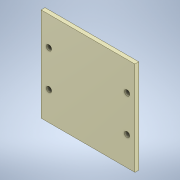
# Autodesk Inventor part: steelPlateForGate
Saved by Autodesk Inventor 2020 (Build 240168000, 168)
## iProperties
Created: 2019-07-06
Part Number: steelPlateForGate
Material: Steel, Mild
Document SubType Name: Modeling
Designer: steele
Density: 7.85 g/cm^3
Appearance: Smooth - Ash
Author: steele
Autodesk Inventor part; units mm, degrees
ref_plane "YZ Plane" through (0, 0, 0) normal (1, 0, 0) x (0, 1, 0)
ref_plane "XZ Plane" through (0, 0, 0) normal (0, 1, 0) x (-1, 0, 0)
ref_plane "XY Plane" through (0, 0, 0) normal (0, 0, 1) x (1, 0, 0)
sketch "Sketch1" plane through (0, 0, 0) normal (0, 0, 1) x (1, 0, 0)
  line L0 (-76.2, -76.2) -> (76.2, -76.2)
  line L1 (76.2, -76.2) -> (76.2, 76.2)
  line L2 (76.2, 76.2) -> (-76.2, 76.2)
  line L3 (-76.2, 76.2) -> (-76.2, -76.2)
  line L4 (-76.2, -76.2) -> (76.2, 76.2) construction
  line L5 (76.2, -76.2) -> (-76.2, 76.2) construction
  point P0 (0, 0)
  dimension "d0" = 152.4
  dimension "d1" = 152.4
  constraints: 12 end point, 2 midpoint, 2 parallel, 1 horizontal, 1 perpendicular
  measures "d0" distance of L0.start L0.end
  measures "d1" distance of L1.end L0.end
extrude "Extrusion1" add sketch "Sketch1" along normal blind 6.35
sketch "Sketch2" plane through (0, 0, 6.35) normal (0, 0, 1) x (1, 0, 0)
  line L0 (-63.5, -29.3688) -> (63.5, -29.3688) construction
  line L1 (63.5, -29.3688) -> (63.5, 29.3688) construction
  line L2 (63.5, 29.3688) -> (-63.5, 29.3687) construction
  line L3 (-63.5, 29.3687) -> (-63.5, -29.3688) construction
  line L4 (-63.5, -29.3688) -> (63.5, 29.3688) construction
  line L5 (63.5, -29.3688) -> (-63.5, 29.3687) construction
  point P0 (0, 0)
  dimension "d4" = 127
  dimension "d5" = 58.7375
  constraints: 12 end point, 4 coincident, 2 midpoint, 2 parallel, 1 horizontal, 1 perpendicular
  measures "d4" distance of L0.start L0.end
  measures "d5" distance of L2.end L0.start
hole "Hole1" at (-63.5, 29.3687, 6.35) at (63.5, 29.3688, 6.35) at (63.5, -29.3688, 6.35) at (-63.5, -29.3688, 6.35) direction (0, 0, -1) diameter 8.7376 end through all clearance for "Flat Head Machine Screw (82)" size "5/16" standard "Ansi Unified Screw Threads"
body "Solid1"
